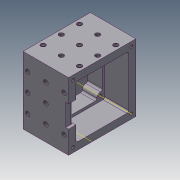
# Autodesk Inventor part: J005679
Saved by Autodesk Inventor 2015 SP1 (Build 190203100, 203)
## iProperties
Created: 2008-08-14
Part Number: J005679
Document SubType Name: Modeling
Designer: duttaa
Density: 2.71 g/cm^3
Mass: 92.9517 g
Surface Area: 148.088 cm^2
Volume: 34.2995 cm^3
Material: Aluminum-6061
Description: CAMERA FRONT BODY
Vendor: HHMI: JRC - ID&F
Appearance: Aluminum (Flat)
Project: COMMON
ALTERED ITEM DESCRIPTION: N/A
ALTERED ITEM PART NUMBER: N/A
ALTERED ITEM VENDOR: N/A
SPECIAL FINISH: NONE
SURFACE ROUGHNESS: N/A
DESIGN DEPARTMENT: HHMI: JRC - ID&F
LAB/DEPT: COMMON
REQUESTING SCIENTIST: COMMON
Author: duttaa
Autodesk Inventor part; units mm, degrees
note: some values were not read from the file. Chosen so that the rebuilt part matches the saved one: direction of "Hole1".
ref_plane "YZ Plane" through (0, 0, 0) normal (1, 0, 0) x (0, 1, 0)
sketch "Sketch2" plane through (0, 0, 0) normal (1, 0, 0) x (0, 1, 0)
  line L0 (30.0346, 29.5395) -> (-16.9554, 29.5395)
  line L1 (-16.9554, 29.5395) -> (-16.9554, -17.4505)
  line L2 (-16.9554, -17.4505) -> (30.0346, -17.4505)
  line L3 (30.0346, -17.4505) -> (30.0346, 29.5395)
  dimension "d0" = 46.99
  dimension "d1" = 46.99
  constraints: 8 end point, 2 parallel, 1 horizontal, 1 perpendicular
  measures "d0" distance between parallel lines of L2 L0
  measures "d1" distance between parallel lines of L1 L3
extrude "Extrusion1" add sketch "Sketch2" along normal blind 38.1
sketch "Sketch3" plane through (38.1, 0, 0) normal (1, 0, 0) x (0, 0, -1)
  line L0 (-29.5395, 30.0346) -> (17.4505, 30.0346) projected
  line L1 (-29.5395, -16.9554) -> (-29.5395, 30.0346) projected
  line L2 (17.4505, -16.9554) -> (-29.5395, -16.9554) projected
  line L3 (17.4505, 30.0346) -> (17.4505, -16.9554) projected
  line L4 (3.9044, 23.0496) -> (-19.0962, 23.0496)
  line L5 (-22.5545, 19.5912) -> (-22.5545, -3.4094)
  line L6 (-15.9934, -9.9704) -> (7.0072, -9.9704)
  line L7 (10.4655, -6.5121) -> (10.4655, 16.4885)
  arc A0 (-22.5545, 19.5912) -> (-19.0962, 23.0496) centre (-21.3109, 21.806) ccw
  arc A1 (3.9044, 23.0496) -> (10.4655, 16.4885) centre (9.2219, 21.806) ccw
  arc A2 (10.4655, -6.5121) -> (7.0072, -9.9704) centre (9.2219, -8.7269) ccw
  arc A3 (-15.9934, -9.9704) -> (-22.5545, -3.4094) centre (-21.3109, -8.7269) ccw
  line L8 (17.4505, -16.9554) -> (-29.5395, -16.9554) projected
  line L9 (17.4505, 30.0346) -> (17.4505, -16.9554) projected
  line L10 (-6.0445, 27.4855) -> (-6.0445, -19.3274)
  line L11 (-28.3078, 6.5396) -> (17.8192, 6.5396)
  line L12 (-21.3109, 21.806) -> (9.2219, -8.7269)
  line L13 (-21.3109, -8.7269) -> (9.2219, 21.806)
  dimension "d42" = 2.54
  dimension "d49" = 46.99
  dimension "d50" = 23.495
  dimension "d51" = 46.99
  dimension "d52" = 23.495
  dimension "d68" = 43.18
  dimension "d69" = 43.18
  dimension "d78" = 5.461
  dimension "d79" = 5.461
  dimension "d80" = 2.54
  dimension "d84" = 33.02
  dimension "d85" = 33.02
  constraints: 16 end point, 8 point on circle, 4 centre point, 3 parallel, 3 symmetric about line, 2 perpendicular
  measures "d42" radius of A0
  measures "d49" distance between parallel lines of L3 L1
  measures "d50" distance between parallel lines of L10 L1
  measures "d51" distance between parallel lines of L8 L0
  measures "d52" distance between parallel lines of L11 L0
  measures "d68" distance of L12.end L12.start
  measures "d69" distance of L13.end L13.start
  measures "d78" radius of A1
  measures "d79" radius of A3
  measures "d80" radius of A2
  measures "d84" distance between parallel lines of L6 L4
  measures "d85" distance between parallel lines of L7 L5
extrude "Extrusion2" cut sketch "Sketch3" against normal blind 33.02 contours L11 L13 A1 L7 | L7 A2 L12 L11 | L10 L12 A2 L6 | L6 A3 L13 L10 | L12 A0 L4 L10 | L13 A3 L5 L11 | L11 L5 A0 L12 | L10 L4 A1 L13
sketch "Sketch4" plane through (0, 0, 0) normal (-1, 0, 0) x (0, 0, 1)
  line L0 (29.5395, 30.0346) -> (29.5395, -16.9554) projected
  line L1 (-17.4505, 30.0346) -> (29.5395, 30.0346) projected
  line L2 (-17.4505, -16.9554) -> (-17.4505, 30.0346) projected
  line L3 (29.5395, -16.9554) -> (-17.4505, -16.9554) projected
  line L4 (-19.6876, 6.5396) -> (25.2381, 6.5396)
  line L5 (6.0445, 23.3198) -> (6.0445, -18.8213)
  point P0 (6.0445, 6.5396)
  dimension "d7" = 46.99
  dimension "d8" = 23.495
  dimension "d9" = 46.99
  dimension "d10" = 23.495
  constraints: 4 end point, 2 point on line, 1 parallel, 1 perpendicular
  measures "d7" distance between parallel lines of L0 L2
  measures "d8" distance between parallel lines of L5 L2
  measures "d9" distance between parallel lines of L3 L1
  measures "d10" distance between parallel lines of L4 L1
hole "Hole1" at (0, 6.5396, 6.0445) direction (1, 0, 0) diameter 24.5364 end up to surface thread size "1-32 UN" class "2B" standard "ANSI Unified Screw Threads"
sketch "Sketch5" plane through (38.1, 0, 0) normal (1, 0, 0) x (0, 0, -1)
  line L0 (-29.5395, 30.0346) -> (17.4505, 30.0346) projected
  line L1 (-29.5395, -16.9554) -> (-29.5395, 30.0346) projected
  line L2 (17.4505, -16.9554) -> (-29.5395, -16.9554) projected
  line L3 (17.4505, 30.0346) -> (17.4505, -16.9554) projected
  line L4 (12.3705, 24.9546) -> (-24.4595, 24.9546)
  line L5 (-24.4595, 24.9546) -> (-24.4595, -11.8754)
  line L6 (-24.4595, -11.8754) -> (12.3705, -11.8754)
  line L7 (12.3705, -11.8754) -> (12.3705, 24.9546)
  circle A0 centre (-6.0445, 6.5396) radius 12.2682 projected
  dimension "d90" = 36.83
  dimension "d91" = 36.83
  dimension "d92" = 18.415
  dimension "d93" = 18.415
  constraints: 8 end point, 3 other
  measures "d90" distance between parallel lines of L6 L4
  measures "d91" distance between parallel lines of L7 L5
  measures "d92" distance from line of L4 A0.centre
  measures "d93" distance from line of L5 A0.centre
extrude "Extrusion3" cut sketch "Sketch5" against normal blind 22.86 contours L7 L6 L5 L4 | A0
sketch "Sketch6" plane through (15.24, 0, 0) normal (1, 0, 0) x (0, 0, -1)
  line L0 (-24.4595, 24.9546) -> (-24.4595, -11.8754) projected
  line L1 (12.3705, 24.9546) -> (-24.4595, 24.9546) projected
  line L2 (12.3705, -11.8754) -> (12.3705, 24.9546) projected
  line L3 (-24.4595, -11.8754) -> (12.3705, -11.8754) projected
  arc A0 (3.9044, 23.0496) -> (10.4655, 16.4885) centre (9.2219, 21.806) ccw projected
  arc A1 (10.4655, -6.5121) -> (7.0072, -9.9704) centre (9.2219, -8.7269) ccw projected
  arc A2 (-15.9934, -9.9704) -> (-22.5545, -3.4094) centre (-21.3109, -8.7269) ccw projected
  arc A3 (-22.5545, 19.5912) -> (-19.0962, 23.0496) centre (-21.3109, 21.806) ccw projected
  dimension "d70" = 43.18
  dimension "d71" = 43.18
  constraints: 4 coincident
  measures "d70" distance of A1.centre A3.centre
  measures "d71" distance of A0.centre A2.centre
hole "Hole3" at (15.24, 21.806, 21.3109) at (15.24, 21.806, -9.2219) at (15.24, -8.7269, -9.2219) at (15.24, -8.7269, 21.3109) direction (-1, 0, 0) diameter 2.159 depth 12.7 tip angle 118
fillet "Fillet1" radius 1.27 8 edges at (10.16, 19.5912, 22.5545) (10.16, 23.0496, 19.0962) (10.16, 23.0496, -3.9044) (10.16, 16.4885, -10.4655) (10.16, -6.5121, -10.4655) (10.16, -3.4094, 22.5545) (10.16, -9.9704, 15.9934) (10.16, -9.9704, -7.0072)
sketch "Sketch7" plane through (15.24, 0, 0) normal (1, 0, 0) x (0, 0, -1)
  arc A0 (9.2043, -6.1869) -> (6.682, -8.7093) centre (9.2219, -8.7269) ccw projected
  arc A1 (-15.85, -8.7054) -> (-21.2895, -3.2659) centre (-21.3109, -8.7269) ccw projected
  arc A2 (-21.2933, 19.2661) -> (-18.771, 21.7884) centre (-21.3109, 21.806) ccw projected
  arc A3 (3.761, 21.7845) -> (9.2005, 16.345) centre (9.2219, 21.806) ccw projected
  line L0 (-21.3109, -8.7269) -> (9.2219, 21.806)
  line L1 (-21.3109, 21.806) -> (9.2219, -8.7269)
  circle A4 centre (-18.078, -5.494) radius 0.762
  circle A5 centre (-6.0445, 6.5396) radius 12.2682 projected
  circle A6 centre (5.989, 18.5731) radius 0.762
  dimension "d94" = 1.524
  dimension "d95" = 17.018
  constraints: 4 end point, 2 centre point, 1 perpendicular, 1 point on line, 1 symmetric about line, 1 other
  measures "d94" diameter of A4
  measures "d95" distance of A5.centre A4.centre
extrude "Extrusion4" add sketch "Sketch7" along normal blind 1.27 contours A4 L0 | L0 A4 | A6 L0 | L0 A6
sketch "Sketch8" plane through (0, -16.9554, -17.4505) normal (0, 0, -1) x (-1, 0, 0)
  line L0 (0, 0) -> (0, 46.99) projected
  line L1 (-43.6773, 47.131) -> (-31.75, 47.131)
  line L2 (-31.75, 47.131) -> (-31.75, -4.1884)
  line L3 (-31.75, -4.1884) -> (-43.6773, -4.1884)
  line L4 (-43.6773, -4.1884) -> (-43.6773, 47.131)
  dimension "d81" = 31.75
  constraints: 8 end point, 2 parallel, 1 horizontal, 1 perpendicular
  measures "d81" distance between parallel lines of L0 L2
extrude "Extrusion5" cut sketch "Sketch8" against normal through all
fillet "Fillet2" radius 1.27 4 edges at (23.495, 24.9546, 24.4595) (23.495, 24.9546, -12.3705) (23.495, -11.8754, 24.4595) (23.495, -11.8754, -12.3705)
sketch "Sketch9" plane through (31.75, -16.9554, -17.4505) normal (1, 0, 0) x (0, 0, -1)
  line L0 (0, 0) -> (-46.99, 0) projected
  line L1 (0, 46.99) -> (0, 0) projected
  line L2 (-46.99, 46.99) -> (0, 46.99) projected
  line L3 (-46.99, 0) -> (-46.99, 46.99) projected
  line L4 (-41.91, 40.64) -> (-41.91, 6.35) projected
  line L5 (-23.495, 43.4944) -> (-23.495, -1.6796)
  line L6 (-48.0819, 23.495) -> (4.574, 23.495)
  point P0 (-43.815, 43.815)
  point P1 (-3.175, 43.815)
  point P2 (-3.175, 3.175)
  point P3 (-43.815, 3.175)
  dimension "d97" = 23.495
  dimension "d98" = 46.99
  dimension "d99" = 23.495
  dimension "d100" = 46.99
  dimension "d101" = 40.64
  dimension "d102" = 40.64
  constraints: 4 end point, 3 symmetric about line, 1 parallel, 1 perpendicular
  measures "d97" distance between parallel lines of L5 L3
  measures "d98" distance between parallel lines of L1 L3
  measures "d99" distance between parallel lines of L6 L2
  measures "d100" distance between parallel lines of L0 L2
  measures "d101" distance of point (-3.175, 43.815) point (-43.815, 43.815)
  measures "d102" distance of point (-43.815, 3.175) point (-43.815, 43.815)
hole "Hole4" at (31.75, 26.8596, 26.3645) at (31.75, 26.8596, -14.2755) at (31.75, -13.7804, -14.2755) at (31.75, -13.7804, 26.3645) direction (-1, 0, 0) diameter 2.159 depth 12.7 tip angle 118
sketch "Sketch10" plane through (31.75, -16.9554, -17.4505) normal (1, 0, 0) x (0, 0, -1)
  line L0 (0, 0) -> (-46.99, 0) projected
  line L1 (0, 46.99) -> (0, 0) projected
  line L2 (-46.99, 46.99) -> (0, 46.99) projected
  line L3 (-46.99, 0) -> (-46.99, 46.99) projected
  line L4 (-41.91, 40.64) -> (-41.91, 6.35) projected
  line L5 (-53.1634, 23.495) -> (4.5275, 23.495)
  line L6 (-23.495, 45.4708) -> (-23.495, -1.162)
  line L7 (-46.99, 31.115) -> (-41.91, 31.115)
  line L8 (-46.99, 15.875) -> (-41.91, 15.875)
  dimension "d110" = 46.99
  dimension "d111" = 23.495
  dimension "d112" = 46.99
  dimension "d113" = 23.495
  dimension "d114" = 15.24
  constraints: 8 end point, 4 perpendicular, 4 point on line, 2 symmetric about line
  measures "d110" distance between parallel lines of L1 L3
  measures "d111" distance between parallel lines of L6 L3
  measures "d112" distance between parallel lines of L0 L2
  measures "d113" distance between parallel lines of L5 L2
  measures "d114" distance between parallel lines of L8 L7
extrude "Extrusion6" cut sketch "Sketch10" against normal blind 1.905 contours L3 L5 L4 L8 | L5 L3 L7 L4
sketch "Sketch11" plane through (0, -16.9554, 29.5395) normal (0, 0, 1) x (1, 0, 0)
  line L0 (31.75, 31.115) -> (31.75, 46.99) projected
  line L1 (0, 46.99) -> (31.75, 46.99) projected
  line L2 (0, 46.99) -> (0, 0) projected
  line L3 (0, 0) -> (31.75, 0) projected
  line L4 (0.2116, 23.495) -> (39.1885, 23.495)
  line L5 (15.875, 50.9583) -> (15.875, -3.977)
  line L6 (29.845, 15.875) -> (29.845, 31.115) projected
  line L7 (3.175, 36.195) -> (28.575, 36.195)
  line L8 (28.575, 36.195) -> (28.575, 10.795)
  line L9 (28.575, 10.795) -> (3.175, 10.795)
  line L10 (3.175, 10.795) -> (3.175, 36.195)
  point P0 (15.875, 36.195)
  point P1 (3.175, 23.495)
  point P2 (15.875, 10.795)
  point P3 (15.875, 23.4906)
  point P4 (28.575, 23.495)
  dimension "d117" = 31.75
  dimension "d120" = 46.99
  dimension "d121" = 23.495
  dimension "d131" = 15.875
  dimension "d132" = 25.4
  dimension "d133" = 25.4
  constraints: 12 end point, 5 midpoint, 3 symmetric about line, 2 parallel, 2 perpendicular
  measures "d117" distance between parallel lines of L0 L2
  measures "d120" distance between parallel lines of L3 L1
  measures "d121" distance between parallel lines of L4 L1
  measures "d131" distance between parallel lines of L5 L2
  measures "d132" distance of L7.end L7.start
  measures "d133" distance of L9.end L7.start
hole "Hole6" at (3.175, 19.2396, 29.5395) at (28.575, 19.2396, 29.5395) at (28.575, -6.1604, 29.5395) at (3.175, -6.1604, 29.5395) at (15.875, 19.2396, 29.5395) at (3.175, 6.5396, 29.5395) at (15.875, 6.5352, 29.5395) at (15.875, -6.1604, 29.5395) direction (0, 0, -1) diameter 3.302 depth 4.064 thread size "8-32 UNC" class "2B" standard "ANSI Unified Screw Threads"
ref_plane "Work Plane1" through (76.6011, 6.5396, 6.0445) normal (0, 0, -1) x (-1, 0, 0)
mirror "Mirror1" about plane through (76.6011, 6.5396, 6.0445) normal (0, 0, -1) of "Hole6"
sketch "Sketch12" plane through (0, 30.0346, 29.5395) normal (0, 1, 0) x (1, 0, 0)
  line L0 (31.75, 0) -> (31.75, 46.99) projected
  line L1 (0, 46.99) -> (31.75, 46.99) projected
  line L2 (0, 46.99) -> (0, 0) projected
  line L3 (0, 0) -> (31.75, 0) projected
  line L4 (15.875, 52.0718) -> (15.875, -3.5778)
  line L5 (-5.1132, 23.495) -> (37.752, 23.495)
  line L6 (3.175, 36.195) -> (3.175, 10.795)
  line L7 (3.175, 10.795) -> (28.575, 10.795)
  line L8 (28.575, 10.795) -> (28.575, 36.195)
  line L9 (28.575, 36.195) -> (3.175, 36.195)
  point P0 (15.875, 36.195)
  point P1 (3.175, 23.495)
  point P2 (15.875, 10.795)
  point P3 (28.575, 23.495)
  point P4 (15.875, 23.495)
  dimension "d142" = 31.75
  dimension "d143" = 15.875
  dimension "d144" = 46.99
  dimension "d145" = 23.495
  dimension "d146" = 25.4
  dimension "d147" = 25.4
  constraints: 12 end point, 6 point on line, 4 midpoint, 4 perpendicular, 3 symmetric about line, 2 parallel
  measures "d142" distance between parallel lines of L0 L2
  measures "d143" distance between parallel lines of L4 L2
  measures "d144" distance between parallel lines of L3 L1
  measures "d145" distance between parallel lines of L5 L1
  measures "d146" distance of L8.end L6.start
  measures "d147" distance of L6.end L6.start
hole "Hole7" at (3.175, 30.0346, -6.6555) at (28.575, 30.0346, -6.6555) at (28.575, 30.0346, 18.7445) at (3.175, 30.0346, 18.7445) at (15.875, 30.0346, -6.6555) at (3.175, 30.0346, 6.0445) at (15.875, 30.0346, 18.7445) at (15.875, 30.0346, 6.0445) at (28.575, 30.0346, 6.0445) direction (0, -1, 0) diameter 3.302 depth 4.064 thread size "8-32 UNC" class "2B" standard "ANSI Unified Screw Threads"
ref_plane "Work Plane2" through (76.6011, 6.5396, 6.0445) normal (0, 1, 0) x (-1, 0, 0)
mirror "Mirror2" about plane through (76.6011, 6.5396, 6.0445) normal (0, 1, 0) of "Hole7"
fillet "Fillet4" radius 1.5875 1 edges at (29.845, 6.5396, 24.4595)
equation "\"d0\" = d1"
equation "\"d50\" = 0.5 * d49"
equation "\"d52\" = 0.5 * d51"
equation "\"d78\" = d79"
equation "\"d80\" = d42"
equation "\"d8\" = 0.5 * d7"
equation "\"d10\" = 0.5 * d9"
equation "\"d97\" = 0.5 * d98"
equation "\"d99\" = 0.5 * d100"
equation "\"d101\" = d102"
equation "\"d111\" = 0.5 * d110"
equation "\"d113\" = 0.5 * d112"
equation "\"d121\" = 0.5 * d120"
equation "\"d131\" = 0.5 * d117"
equation "\"d143\" = 0.5 * d142"
equation "\"d145\" = 0.5 * d144"
body "Solid1"
